# Autodesk Inventor part: PAS-PHOENIXTERMINAL2PIN-10_16MM
Saved by Autodesk Inventor 2016 (Build 200138000, 138)
## iProperties
Created: 2016-04-08
Part Number: PAS-PHOENIXTERMINAL2PIN-10_16MM
Material: Generic
Document SubType Name: Modeling
Designer: Paschalis
Density: 1 g/cm^3
Appearance: PAS-PHOENIXTERMINAL-2PIN-10_16MM, PAS-PHOENIXTERMINAL2PIN-10_16MM
Author: Paschalis
Autodesk Inventor part; units mm, degrees
ref_plane "YZ Plane" through (0, 0, 0) normal (1, 0, 0) x (0, 1, 0)
ref_plane "XZ Plane" through (0, 0, 0) normal (0, 1, 0) x (-1, 0, 0)
ref_plane "XY Plane" through (0, 0, 0) normal (0, 0, 1) x (1, 0, 0)
sketch3d "PAS-PHOENIXTERMINAL-2PIN-10_16MM, PAS-PHOENIXTERMINAL2PIN-10"
  constraints: 8 end point
sketch "PAS-PHOENIXTERMINAL-2PIN-10_16MM, PAS-PHOENIXTERMINAL2PIN-10_16MM_123" plane through (0, 0, 0) normal (0, 0, 1) x (1, 0, 0)
  line L0 (-10.3235, 9.2635) -> (10.3235, 9.2635)
  line L1 (10.3235, 9.2635) -> (10.3235, -9.2)
  line L2 (10.3235, -9.2) -> (-10.3235, -9.2)
  line L3 (-10.3235, -9.2) -> (-10.3235, 9.2635)
extrude "Extrusion1" add sketch "PAS-PHOENIXTERMINAL-2PIN-10_16MM, PAS-PHOENIXTERMINAL2PIN-10_16MM_123" along normal blind 1
body "Solid1"
